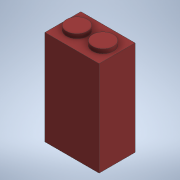
# Autodesk Inventor part: PowerSource
Saved by Autodesk Inventor 2021 (Build 250183000, 183)
## iProperties
Created: 2021-01-19
Part Number: PowerSource
Material: Generic
Document SubType Name: Modeling
Designer: Jayan
Density: 1 g/cm^3
Appearance: Default
Author: Jayan
Autodesk Inventor part; units mm, degrees
ref_plane "YZ Plane" through (0, 0, 0) normal (1, 0, 0) x (0, 1, 0)
ref_plane "XZ Plane" through (0, 0, 0) normal (0, 1, 0) x (-1, 0, 0)
ref_plane "XY Plane" through (0, 0, 0) normal (0, 0, 1) x (1, 0, 0)
sketch "Sketch1" plane through (0, 0, 0) normal (0, 0, 1) x (1, 0, 0)
  line L0 (0, 0) -> (26.416, 0)
  line L1 (26.416, 0) -> (26.416, 46.228)
  line L2 (26.416, 46.228) -> (0, 46.228)
  line L3 (0, 46.228) -> (0, 0)
  dimension "d0" = 26.416
  dimension "d1" = 46.228
  constraints: 8 end point, 2 parallel, 1 horizontal, 1 perpendicular
  measures "d0" distance of L2.end L1.end
  measures "d1" distance of L1.end L0.end
extrude "Extrusion1" add sketch "Sketch1" along normal blind 17.526
sketch "Sketch2" plane through (0, 46.228, 0) normal (0, 1, 0) x (1, 0, 0)
  line L0 (26.416, 0) -> (0, 0) projected
  line L1 (0, 0) -> (6.858, 0)
  line L2 (26.416, 0) -> (19.558, 0)
  line L3 (6.858, 0) -> (6.858, -8.763)
  line L4 (19.558, 0) -> (19.558, -8.763)
  line L5 (6.858, -8.763) -> (19.558, -8.763)
  circle A0 centre (6.858, -8.763) radius 5.08
  circle A1 centre (19.558, -8.763) radius 5.08
  dimension "d4" = 6.858
  dimension "d5" = 6.858
  dimension "d6" = 8.763
  dimension "d7" = 8.763
  dimension "d8" = 10.16
  dimension "d9" = 10.16
  constraints: 10 end point, 2 centre point, 2 coincident, 2 point on line, 2 vertical
  measures "d4" distance of L0.end L1.end
  measures "d5" distance of L0.start L2.end
  measures "d6" distance of L1.end L3.end
  measures "d7" distance of L2.end L4.end
  measures "d8" diameter of A0
  measures "d9" diameter of A1
extrude "Extrusion2" add sketch "Sketch2" along normal blind 2.032 contours A1 L5 L4 | L4 L5 A1 | A0 L5 L3 | L3 L5 A0
body "Solid1"
